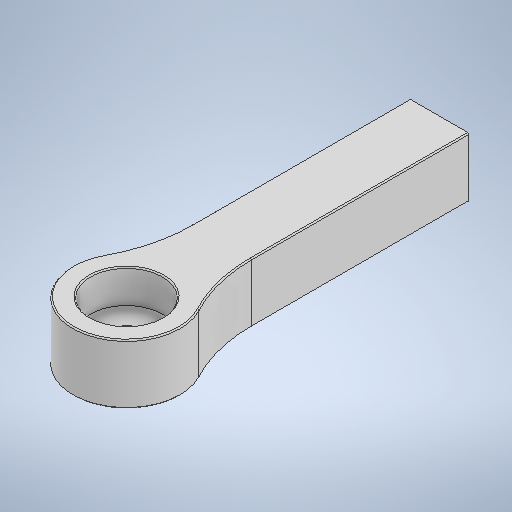
# Autodesk Inventor part: alternativeJoint2
Saved by Autodesk Inventor 2025.1 (Build 291241000, 241)
## iProperties
Created: 2024-11-07
Part Number: alternativeJoint2
Material: Generisch
Document SubType Name: Modeling
Designer: ZOMBULLI
Density: 1 g/cm^3
Appearance: Vorgabe
Author: ZOMBULLI
Autodesk Inventor part; units mm, degrees
ref_plane "YZ Plane" through (0, 0, 0) normal (1, 0, 0) x (0, 1, 0)
ref_plane "XZ Plane" through (0, 0, 0) normal (0, 1, 0) x (-1, 0, 0)
ref_plane "XY Plane" through (0, 0, 0) normal (0, 0, 1) x (1, 0, 0)
sketch "Skizze1" plane through (0, 0, 0) normal (0, 0, 1) x (1, 0, 0)
  line L0 (5, 52.5) -> (-5, 52.5)
  line L1 (-5, 52.5) -> (-5, 16)
  line L2 (5, 16) -> (5, 52.5)
  arc A0 (-7.9412, 4.2353) -> (7.9412, 4.2353) centre (0, 0) ccw
  arc A1 (5, 16) -> (7.9412, 4.2353) centre (30, 16) ccw
  arc A2 (-7.9412, 4.2353) -> (-5, 16) centre (-30, 16) ccw
  line L3 (0, -25.0931) -> (0, 22.9698)
  line L4 (0, 68.0186) -> (0, -40.6118) projected
  point P0 (0, 0)
  point P1 (0, 0)
  point P2 (-5, 7.4833)
  point P3 (5, 7.4833)
  dimension "d1" = 18
  dimension "d4" = 25
  dimension "d7" = 0
  dimension "d8" = 52.5
  dimension "d9" = 0
  dimension "d10" = 0
  dimension "d20" = 5
  dimension "d21" = 5
  constraints: 8 end point, 8 point on circle, 4 tangent, 3 centre point, 2 point on line, 1 equal radius, 1 horizontal, 1 parallel, 1 perpendicular
  measures "d1" diameter of A0
  measures "d4" radius of A2
  measures "d7" distance of A0.centre point (0, 0)
  measures "d8" distance from line of point (0, 0) L0
  measures "d9" distance between parallel lines of L4 L3
  measures "d10" distance of point (0, 0) point (0, 0)
  measures "d20" distance between parallel lines of L4 L1
  measures "d21" distance between parallel lines of L4 L2
extrude "Extrusion1" add sketch "Skizze1" along normal blind 10
sketch "Skizze4" plane through (0, 0, 10) normal (0, 0, 1) x (1, 0, 0)
  circle A0 centre (0, 0) radius 6.05
  dimension "d22" = 12.1
  constraints: 1 centre point, 1 coincident
  measures "d22" diameter of A0
extrude "Extrusion2" cut sketch "Skizze4" against normal blind 5.6
fillet "Rundung1" radius 0.2 1 edges at (-6.05, 0, 10)
fillet "Rundung2" radius 0.2 10 edges at (5, 34.25, 10) (0, -9, 10) (-5.7464, 9.9366, 10) (-5, 34.25, 10) (5.7464, 9.9366, 10) (5, 34.25, 0) (0, -9, 0) (-5.7464, 9.9366, 0) (-5, 34.25, 0) (5.7464, 9.9366, 0)
sketch "Skizze5" plane through (0, 0, 0) normal (0, 0, -1) x (-1, 0, 0)
  circle A0 centre (0, 0) radius 1.75
  dimension "d27" = 3.5
  constraints: 1 centre point, 1 coincident
  measures "d27" diameter of A0
extrude "Extrusion3" cut sketch "Skizze5" against normal up to next
fillet "Rundung3" radius 0.2 2 edges at (1.75, 0, 0) (1.75, 0, 4.4)
sketch "Skizze6" plane through (-4.8, 52.5, 0) normal (0, 1, 0) x (1, 0, 0)
  circle A0 centre (4.8, -5) radius 1.75
  line L0 (9.6, -10) -> (0, -10) projected
  line L1 (9.8, -0.2) -> (9.8, -9.8) projected
  point P0 (4.8, 0)
  dimension "d31" = 3.5
  dimension "d32" = 5
  dimension "d33" = 5
  constraints: 1 centre point
  measures "d31" diameter of A0
  measures "d32" distance from line of L0 A0.centre
  measures "d33" distance from line of A0.centre L1
extrude "Extrusion4" cut sketch "Skizze6" against normal blind 4
sketch "Skizze7" plane through (0, 0, 0) normal (0, 0, -1) x (-1, 0, 0)
  circle A0 centre (0, 0) radius 4
  dimension "d36" = 8
  constraints: 1 centre point, 1 coincident
  measures "d36" diameter of A0
extrude "Extrusion5" cut sketch "Skizze7" against normal blind 3
